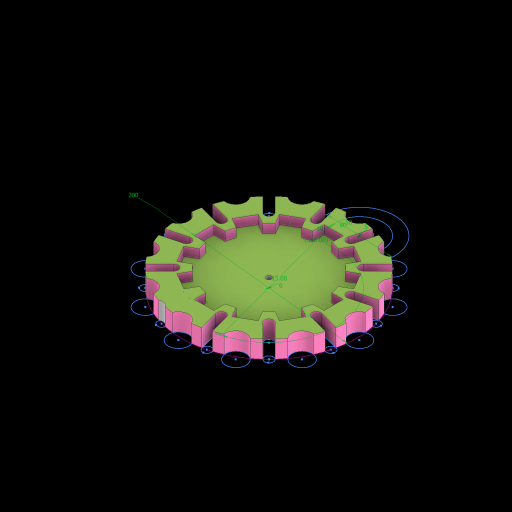
# Autodesk Inventor part: Geneva Gear 12
Saved by Autodesk Inventor 2023 (Build 270158000, 158)
## iProperties
Created: 2022-10-22
Part Number: Geneva Gear 12
Material: Generic
Document SubType Name: Modeling
Designer: annah
Density: 1 g/cm^3
Appearance: Default
Author: annah
Autodesk Inventor part; units mm, degrees
ref_plane "YZ Plane" through (0, 0, 0) normal (1, 0, 0) x (0, 1, 0)
ref_plane "XZ Plane" through (0, 0, 0) normal (0, 1, 0) x (-1, 0, 0)
ref_plane "XY Plane" through (0, 0, 0) normal (0, 0, 1) x (1, 0, 0)
sketch "Sketch1" plane through (0, 0, 0) normal (0, 1, 0) x (-1, 0, 0)
  line L0 (19.134172, -46.193977) -> (0, -54.123064)
  line L1 (0, -54.123064) -> (0, 0)
  line L2 (0, 0) -> (19.134172, -46.193977)
  circle A0 centre (0, 0) radius 50
  line L3 (17.249136, -28.614096) -> (23.883792, -44.631571)
  circle A1 centre (0, -54.123064) radius 20.712
  arc A2 (17.535481, -29.305393) -> (8.166463, -32.781215) centre (12.785861, -30.867798) ccw
  line L4 (14.515069, -48.108105) -> (8.166463, -32.781215)
  line L5 (19.134172, -41.193977) -> (0, -41.193977)
  circle A3 centre (0, -54.123064) radius 12.929087
  arc A4 (-11.696069, -48.612776) -> (11.696069, -48.612776) centre (0, 0) ccw
  arc A5 (-11.696069, -48.612776) -> (11.696069, -48.612776) centre (0, -54.123064) ccw
  circle A6 centre (0, -54.123064) radius 32.5
  arc A7 (19.134172, -41.193977) -> (16.676498, -41.839687) centre (19.134172, -46.193977) ccw
  arc A8 (14.424881, -47.874031) -> (23.597447, -43.940275) centre (19.134172, -46.193977) ccw
  line L6 (32.430202, -8.03624) -> (48.447678, -14.670896)
  arc A9 (33.1215, -8.322585) -> (28.954381, -17.405258) centre (30.867798, -12.785861) ccw
  line L7 (44.281271, -23.753864) -> (28.954381, -17.405258)
  arc A10 (44.051983, -23.652121) -> (47.756382, -14.384552) centre (46.193977, -19.134172) ccw
  circle A11 centre (38.270785, -38.270785) radius 12.929087
  line L8 (28.614096, 17.249136) -> (44.631571, 23.883792)
  arc A12 (29.305393, 17.535481) -> (32.781215, 8.166463) centre (30.867798, 12.785861) ccw
  line L9 (48.108105, 14.515069) -> (32.781215, 8.166463)
  arc A13 (47.874031, 14.424881) -> (43.940275, 23.597447) centre (46.193977, 19.134172) ccw
  circle A14 centre (54.123064, 0) radius 12.929087
  line L10 (8.03624, 32.430202) -> (14.670896, 48.447678)
  arc A15 (8.322585, 33.1215) -> (17.405258, 28.954381) centre (12.785861, 30.867798) ccw
  line L11 (23.753864, 44.281271) -> (17.405258, 28.954381)
  arc A16 (23.652121, 44.051983) -> (14.384552, 47.756382) centre (19.134172, 46.193977) ccw
  circle A17 centre (38.270785, 38.270785) radius 12.929087
  line L12 (-17.249136, 28.614096) -> (-23.883792, 44.631571)
  arc A18 (-17.535481, 29.305393) -> (-8.166463, 32.781215) centre (-12.785861, 30.867798) ccw
  line L13 (-14.515069, 48.108105) -> (-8.166463, 32.781215)
  arc A19 (-14.424881, 47.874031) -> (-23.597447, 43.940275) centre (-19.134172, 46.193977) ccw
  circle A20 centre (0, 54.123064) radius 12.929087
  line L14 (-32.430202, 8.03624) -> (-48.447678, 14.670896)
  arc A21 (-33.1215, 8.322585) -> (-28.954381, 17.405258) centre (-30.867798, 12.785861) ccw
  line L15 (-44.281271, 23.753864) -> (-28.954381, 17.405258)
  arc A22 (-44.051983, 23.652121) -> (-47.756382, 14.384552) centre (-46.193977, 19.134172) ccw
  circle A23 centre (-38.270785, 38.270785) radius 12.929087
  line L16 (-28.614096, -17.249136) -> (-44.631571, -23.883792)
  arc A24 (-29.305393, -17.535481) -> (-32.781215, -8.166463) centre (-30.867798, -12.785861) ccw
  line L17 (-48.108105, -14.515069) -> (-32.781215, -8.166463)
  arc A25 (-47.874031, -14.424881) -> (-43.940275, -23.597447) centre (-46.193977, -19.134172) ccw
  circle A26 centre (-54.123064, 0) radius 12.929087
  line L18 (-8.03624, -32.430202) -> (-14.670896, -48.447678)
  arc A27 (-8.322585, -33.1215) -> (-17.405258, -28.954381) centre (-12.785861, -30.867798) ccw
  line L19 (-23.753864, -44.281271) -> (-17.405258, -28.954381)
  arc A28 (-23.652121, -44.051983) -> (-14.384552, -47.756382) centre (-19.134172, -46.193977) ccw
  circle A29 centre (-38.270785, -38.270785) radius 12.929087
  circle A30 centre (0, 0) radius 3.5
  circle A31 centre (0, -54.123064) radius 3.5
  arc A32 (-7.5, -54.123064) -> (7.5, -54.123064) centre (0, -54.123064) ccw
  arc A33 (7.5, 0) -> (-7.5, 0) centre (0, 0) ccw
  line L20 (7.5, 0) -> (7.5, -54.123064)
  line L21 (-7.5, 0) -> (-7.5, -54.123064)
  circle A34 centre (0, -33.411064) radius 5
  point P0 (8.166168, -32.780503)
  point P1 (23.597447, -43.940275)
  point P2 (28.953669, -17.404963)
  point P3 (29.12854, -29.12854)
  point P4 (26.104054, -42.644793)
  point P5 (42.644793, -26.104054)
  point P6 (32.780503, 8.166168)
  point P7 (41.193977, 0)
  point P8 (48.612776, -11.696069)
  point P9 (48.612776, 11.696069)
  point P10 (17.404963, 28.953669)
  point P11 (29.12854, 29.12854)
  point P12 (42.644793, 26.104054)
  point P13 (26.104054, 42.644793)
  point P14 (-8.166168, 32.780503)
  point P15 (0, 41.193977)
  point P16 (11.696069, 48.612776)
  point P17 (-11.696069, 48.612776)
  point P18 (-28.953669, 17.404963)
  point P19 (-29.12854, 29.12854)
  point P20 (-26.104054, 42.644793)
  point P21 (-42.644793, 26.104054)
  point P22 (-32.780503, -8.166168)
  point P23 (-41.193977, 0)
  point P24 (-48.612776, 11.696069)
  point P25 (-48.612776, -11.696069)
  point P26 (-17.404963, -28.953669)
  point P27 (-29.12854, -29.12854)
  point P28 (-42.644793, -26.104054)
  point P29 (-26.104054, -42.644793)
  point P30 (23.652121, -44.051983)
  point P31 (26.104054, -42.644793)
  point P32 (42.644793, -26.104054)
  point P33 (44.049009, -23.657658)
  point P34 (47.874031, -14.424881)
  point P35 (48.612776, -11.696069)
  point P36 (48.612776, 11.696069)
  point P37 (47.875844, 14.418863)
  point P38 (44.051983, 23.652121)
  point P39 (42.644793, 26.104054)
  point P40 (26.104054, 42.644793)
  point P41 (23.657658, 44.049009)
  point P42 (14.424881, 47.874031)
  point P43 (11.696069, 48.612776)
  point P44 (-11.696069, 48.612776)
  point P45 (-14.418863, 47.875844)
  point P46 (-23.652121, 44.051983)
  point P47 (-26.104054, 42.644793)
  point P48 (-42.644793, 26.104054)
  point P49 (-44.049009, 23.657658)
  point P50 (-47.874031, 14.424881)
  point P51 (-48.612776, 11.696069)
  point P52 (-48.612776, -11.696069)
  point P53 (-47.875844, -14.418863)
  point P54 (-44.051983, -23.652121)
  point P55 (-42.644793, -26.104054)
  point P56 (-26.104054, -42.644793)
  point P57 (-23.657658, -44.049009)
  point P58 (-14.424881, -47.874031)
  point P59 (14.418863, -47.875844)
  dimension "d2" = 100
  dimension "d3" = 22.5
  dimension "d4" = 20.712
  dimension "d5" = 50
  dimension "d6" = 54.12306
  dimension "d7" = 10
  dimension "d8" = 25.85817
  dimension "d9" = 65
  dimension "d10" = 360
  dimension "d11" = 7
  dimension "d12" = 7
  dimension "d13" = 15
  dimension "d14" = 15
  dimension "d15" = 10
  constraints: 113 point on circle, 44 end point, 35 centre point, 28 point on line, 9 coincident, 3 tangent, 2 vertical, 1 concentric, 1 parallel, 1 perpendicular, 161 other
  measures "d2" diameter of A0
  measures "d3" angle of L2 L1
  measures "d4" distance of L0.start L0.end
  measures "d5" distance of L1.end L0.start
  measures "d6" distance of L0.end L1.end
  measures "d7" diameter of A2
  measures "d8" diameter of A3
  measures "d9" diameter of A6
  measures "d11" diameter of A30
  measures "d12" diameter of A31
  measures "d13" diameter of A32
  measures "d14" diameter of A33
  measures "d15" diameter of A34
sketch "Sketch2" plane through (0, 0, 0) normal (0, 1, 0) x (-1, 0, 0)
  circle A0 centre (0, 0) radius 100
  line L0 (0, 0) -> (18.565789, -69.288466)
  line L1 (0, 0) -> (0, -103.527618)
  arc A1 (24.644787, -72.667335) -> (14.990656, -75.254151) centre (0, 0) ccw
  circle A2 centre (25.881905, -96.592583) radius 5
  arc A3 (24.729005, -72.981583) -> (15.074653, -75.567772) centre (19.859884, -74.118095) ccw
  line L2 (30.677672, -95.178151) -> (24.644787, -72.667335)
  line L3 (21.052275, -97.886678) -> (14.990656, -75.254151)
  circle A4 centre (0, -103.527618) radius 11.622857
  line L4 (21.052275, -97.886678) -> (25.881905, -96.592583)
  arc A5 (-25.881905, -96.592583) -> (26.719744, -101.521885) centre (0, -103.527618) ccw
  circle A6 centre (0, -103.527618) radius 40
  arc A7 (57.906738, -50.839403) -> (50.838918, -57.906284) centre (54.258212, -54.258212) ccw
  line L5 (67.175144, -74.246212) -> (50.609365, -57.676679)
  line L6 (74.156719, -67.087861) -> (57.676679, -50.609365)
  circle A8 centre (70.710678, -70.710678) radius 5
  circle A9 centre (51.763809, -89.657547) radius 11.622857
  arc A10 (75.568408, -15.074845) -> (72.980936, -24.728854) centre (74.118095, -19.859884) ccw
  line L7 (95.298487, -30.711534) -> (72.667335, -24.644787)
  line L8 (97.765533, -21.021432) -> (75.254151, -14.990656)
  circle A11 centre (96.592583, -25.881905) radius 5
  circle A12 centre (89.657547, -51.763809) radius 11.622857
  arc A13 (72.981583, 24.729005) -> (75.567772, 15.074653) centre (74.118095, 19.859884) ccw
  line L9 (97.886678, 21.052275) -> (75.254151, 14.990656)
  line L10 (95.178151, 30.677672) -> (72.667335, 24.644787)
  circle A14 centre (96.592583, 25.881905) radius 5
  circle A15 centre (103.527618, 0) radius 11.622857
  arc A16 (50.839403, 57.906738) -> (57.906284, 50.838918) centre (54.258212, 54.258212) ccw
  line L11 (74.246212, 67.175144) -> (57.676679, 50.609365)
  line L12 (67.087861, 74.156719) -> (50.609365, 57.676679)
  circle A17 centre (70.710678, 70.710678) radius 5
  circle A18 centre (89.657547, 51.763809) radius 11.622857
  arc A19 (15.074845, 75.568408) -> (24.728854, 72.980936) centre (19.859884, 74.118095) ccw
  line L13 (30.711534, 95.298487) -> (24.644787, 72.667335)
  line L14 (21.021432, 97.765533) -> (14.990656, 75.254151)
  circle A20 centre (25.881905, 96.592583) radius 5
  circle A21 centre (51.763809, 89.657547) radius 11.622857
  arc A22 (-24.729005, 72.981583) -> (-15.074653, 75.567772) centre (-19.859884, 74.118095) ccw
  line L15 (-21.052275, 97.886678) -> (-14.990656, 75.254151)
  line L16 (-30.677672, 95.178151) -> (-24.644787, 72.667335)
  circle A23 centre (-25.881905, 96.592583) radius 5
  circle A24 centre (0, 103.527618) radius 11.622857
  arc A25 (-57.906738, 50.839403) -> (-50.838918, 57.906284) centre (-54.258212, 54.258212) ccw
  line L17 (-67.175144, 74.246212) -> (-50.609365, 57.676679)
  line L18 (-74.156719, 67.087861) -> (-57.676679, 50.609365)
  circle A26 centre (-70.710678, 70.710678) radius 5
  circle A27 centre (-51.763809, 89.657547) radius 11.622857
  arc A28 (-75.568408, 15.074845) -> (-72.980936, 24.728854) centre (-74.118095, 19.859884) ccw
  line L19 (-95.298487, 30.711534) -> (-72.667335, 24.644787)
  line L20 (-97.765533, 21.021432) -> (-75.254151, 14.990656)
  circle A29 centre (-96.592583, 25.881905) radius 5
  circle A30 centre (-89.657547, 51.763809) radius 11.622857
  arc A31 (-72.981583, -24.729005) -> (-75.567772, -15.074653) centre (-74.118095, -19.859884) ccw
  line L21 (-97.886678, -21.052275) -> (-75.254151, -14.990656)
  line L22 (-95.178151, -30.677672) -> (-72.667335, -24.644787)
  circle A32 centre (-96.592583, -25.881905) radius 5
  circle A33 centre (-103.527618, 0) radius 11.622857
  arc A34 (-50.839403, -57.906738) -> (-57.906284, -50.838918) centre (-54.258212, -54.258212) ccw
  line L23 (-74.246212, -67.175144) -> (-57.676679, -50.609365)
  line L24 (-67.087861, -74.156719) -> (-50.609365, -57.676679)
  circle A35 centre (-70.710678, -70.710678) radius 5
  circle A36 centre (-89.657547, -51.763809) radius 11.622857
  arc A37 (-15.074845, -75.568408) -> (-24.728854, -72.980936) centre (-19.859884, -74.118095) ccw
  line L25 (-30.711534, -95.298487) -> (-24.644787, -72.667335)
  line L26 (-21.021432, -97.765533) -> (-14.990656, -75.254151)
  circle A38 centre (-25.881905, -96.592583) radius 5
  circle A39 centre (-51.763809, -89.657547) radius 11.622857
  circle A40 centre (0, 0) radius 3
  circle A41 centre (0, -103.527618) radius 2.5
  point P0 (50.722678, -50.722678)
  point P1 (73.90092, -74.56066)
  point P2 (69.288466, -18.565789)
  point P3 (101.280404, -27.620965)
  point P4 (69.288466, 18.565789)
  point P5 (101.521885, 26.719744)
  point P6 (50.722678, 50.722678)
  point P7 (74.56066, 73.90092)
  point P8 (18.565789, 69.288466)
  point P9 (27.620965, 101.280404)
  point P10 (-18.565789, 69.288466)
  point P11 (-26.719744, 101.521885)
  point P12 (-50.722678, 50.722678)
  point P13 (-73.90092, 74.56066)
  point P14 (-69.288466, 18.565789)
  point P15 (-101.280404, 27.620965)
  point P16 (-69.288466, -18.565789)
  point P17 (-101.521885, -26.719744)
  point P18 (-50.722678, -50.722678)
  point P19 (-74.56066, -73.90092)
  point P20 (-18.565789, -69.288466)
  point P21 (-27.620965, -101.280404)
  point P22 (40.291734, -91.523637)
  point P23 (59.115928, -80.655484)
  point P24 (67.086711, -74.157759)
  point P25 (80.655484, -59.115928)
  point P26 (91.523637, -40.291734)
  point P27 (95.177675, -30.679148)
  point P28 (99.407662, -10.868153)
  point P29 (99.407662, 10.868153)
  point P30 (97.765859, 21.019917)
  point P31 (91.523637, 40.291734)
  point P32 (80.655484, 59.115928)
  point P33 (74.157759, 67.086711)
  point P34 (59.115928, 80.655484)
  point P35 (40.291734, 91.523637)
  point P36 (30.679148, 95.177675)
  point P37 (10.868153, 99.407662)
  point P38 (-10.868153, 99.407662)
  point P39 (-21.019917, 97.765859)
  point P40 (-40.291734, 91.523637)
  point P41 (-59.115928, 80.655484)
  point P42 (-67.086711, 74.157759)
  point P43 (-80.655484, 59.115928)
  point P44 (-91.523637, 40.291734)
  point P45 (-95.177675, 30.679148)
  point P46 (-99.407662, 10.868153)
  point P47 (-99.407662, -10.868153)
  point P48 (-97.765859, -21.019917)
  point P49 (-91.523637, -40.291734)
  point P50 (-80.655484, -59.115928)
  point P51 (-74.157759, -67.086711)
  point P52 (-59.115928, -80.655484)
  point P53 (-40.291734, -91.523637)
  point P54 (-30.679148, -95.177675)
  point P55 (-10.868153, -99.407662)
  point P56 (10.868153, -99.407662)
  point P57 (21.019917, -97.765859)
  dimension "d16" = 200
  dimension "d17" = 15
  dimension "d20" = 10
  dimension "d21" = 10
  dimension "d22" = 80
  dimension "d25" = 360
  dimension "d27" = 6
  dimension "d28" = 5
  constraints: 100 point on circle, 54 end point, 41 centre point, 25 point on line, 8 coincident, 1 vertical, 198 other
  measures "d17" angle of L1 L0
  measures "d20" diameter of A2
  measures "d21" diameter of A3
  measures "d22" diameter of A6
  measures "d27" diameter of A40
  measures "d28" diameter of A41
extrude "Extrusion1" add sketch "Sketch2" along normal blind 20 contours L26 A37 A1 L1 A4 A0 | A0 A6 A1 A37 L25 | A0 A39 L24 A34 A1 A6 | L1 A1 A3 L3 A0 A4 | A37 A6 L1 A1 | A6 A37 A1 | A1 A34 A31 A28 A25 A22 A19 A16 A13 A10 A7 A6 A3 L0 A40 L1 A37 | L1 A6 L0 A3 A1 | A6 A1 A7 L5 A0 A9 | A0 L2 A3 A1 A6 | L1 A40 L0 A6 | A34 L23 A0 A36 L22 A31 A1 | A1 A3 A6 | A6 A3 L0 | A31 L21 A0 A33 L20 A28 A1 | A1 A10 L7 A0 A12 L6 A7 | A28 L19 A0 A30 L18 A25 A1 | A1 A13 L9 A0 A15 L8 A10 | A25 L17 A0 A27 L16 A22 A1 | A1 A16 L11 A0 A18 L10 A13 | A22 L15 A0 A24 L14 A19 A1 | A1 A19 L13 A0 A21 L12 A16 picked at (-24.752418, -72.385942)
sketch "Sketch3" plane through (0, 20, 0) normal (0, 1, 0) x (1, 0, 0)
  circle A0 centre (0, 0) radius 3
  line L0 (-11.003106, 74.096865) -> (11.003106, 74.096865)
  line L1 (11.003106, 74.096865) -> (11.003106, 56.269048)
  line L2 (11.003106, 56.269048) -> (-11.003106, 56.269048)
  line L3 (-11.003106, 56.269048) -> (-11.003106, 74.096865)
  line L4 (11.003106, 74.096865) -> (0, 65.182957) construction
  line L5 (-27.519463, 69.671321) -> (-18.605555, 54.231978)
  line L6 (-18.605555, 54.231978) -> (-37.663494, 43.228872)
  line L7 (-37.663494, 43.228872) -> (-46.577402, 58.668215)
  line L8 (-46.577402, 58.668215) -> (-27.519463, 69.671321)
  line L9 (-58.668215, 46.577402) -> (-43.228872, 37.663494)
  line L10 (-43.228872, 37.663494) -> (-54.231978, 18.605555)
  line L11 (-54.231978, 18.605555) -> (-69.671321, 27.519463)
  line L12 (-69.671321, 27.519463) -> (-58.668215, 46.577402)
  line L13 (-74.096865, 11.003106) -> (-56.269048, 11.003106)
  line L14 (-56.269048, 11.003106) -> (-56.269048, -11.003106)
  line L15 (-56.269048, -11.003106) -> (-74.096865, -11.003106)
  line L16 (-74.096865, -11.003106) -> (-74.096865, 11.003106)
  line L17 (-69.671321, -27.519463) -> (-54.231978, -18.605555)
  line L18 (-54.231978, -18.605555) -> (-43.228872, -37.663494)
  line L19 (-43.228872, -37.663494) -> (-58.668215, -46.577402)
  line L20 (-58.668215, -46.577402) -> (-69.671321, -27.519463)
  line L21 (-46.577402, -58.668215) -> (-37.663494, -43.228872)
  line L22 (-37.663494, -43.228872) -> (-18.605555, -54.231978)
  line L23 (-18.605555, -54.231978) -> (-27.519463, -69.671321)
  line L24 (-27.519463, -69.671321) -> (-46.577402, -58.668215)
  line L25 (-11.003106, -74.096865) -> (-11.003106, -56.269048)
  line L26 (-11.003106, -56.269048) -> (11.003106, -56.269048)
  line L27 (11.003106, -56.269048) -> (11.003106, -74.096865)
  line L28 (11.003106, -74.096865) -> (-11.003106, -74.096865)
  line L29 (27.519463, -69.671321) -> (18.605555, -54.231978)
  line L30 (18.605555, -54.231978) -> (37.663494, -43.228872)
  line L31 (37.663494, -43.228872) -> (46.577402, -58.668215)
  line L32 (46.577402, -58.668215) -> (27.519463, -69.671321)
  line L33 (58.668215, -46.577402) -> (43.228872, -37.663494)
  line L34 (43.228872, -37.663494) -> (54.231978, -18.605555)
  line L35 (54.231978, -18.605555) -> (69.671321, -27.519463)
  line L36 (69.671321, -27.519463) -> (58.668215, -46.577402)
  line L37 (74.096865, -11.003106) -> (56.269048, -11.003106)
  line L38 (56.269048, -11.003106) -> (56.269048, 11.003106)
  line L39 (56.269048, 11.003106) -> (74.096865, 11.003106)
  line L40 (74.096865, 11.003106) -> (74.096865, -11.003106)
  line L41 (69.671321, 27.519463) -> (54.231978, 18.605555)
  line L42 (54.231978, 18.605555) -> (43.228872, 37.663494)
  line L43 (43.228872, 37.663494) -> (58.668215, 46.577402)
  line L44 (58.668215, 46.577402) -> (69.671321, 27.519463)
  line L45 (46.577402, 58.668215) -> (37.663494, 43.228872)
  line L46 (37.663494, 43.228872) -> (18.605555, 54.231978)
  line L47 (18.605555, 54.231978) -> (27.519463, 69.671321)
  line L48 (27.519463, 69.671321) -> (46.577402, 58.668215)
  arc A1 (-11.003106, 60.9667) -> (-20.954381, 58.300264) centre (0, 0) ccw
  arc A2 (20.954381, 58.300264) -> (11.003106, 60.9667) centre (0, 0) ccw
  arc A3 (47.297158, 40.01232) -> (40.01232, 47.297158) centre (0, 0) ccw
  arc A4 (-40.01232, 47.297158) -> (-47.297158, 40.01232) centre (0, 0) ccw
  arc A5 (-58.300264, 20.954381) -> (-60.9667, 11.003106) centre (0, 0) ccw
  arc A6 (-60.9667, -11.003106) -> (-58.300264, -20.954381) centre (0, 0) ccw
  arc A7 (-47.297158, -40.01232) -> (-40.01232, -47.297158) centre (0, 0) ccw
  arc A8 (-20.954381, -58.300264) -> (-11.003106, -60.9667) centre (0, 0) ccw
  arc A9 (11.003106, -60.9667) -> (20.954381, -58.300264) centre (0, 0) ccw
  arc A10 (40.01232, -47.297158) -> (47.297158, -40.01232) centre (0, 0) ccw
  arc A11 (58.300264, -20.954381) -> (60.9667, -11.003106) centre (0, 0) ccw
  arc A12 (60.9667, 11.003106) -> (58.300264, 20.954381) centre (0, 0) ccw
  dimension "d36" = 360
  constraints: 98 end point, 24 point on circle, 24 point on line, 12 centre point, 3 coincident, 2 parallel, 1 horizontal, 1 perpendicular, 97 other
extrude "Extrusion2" cut sketch "Sketch3" against normal blind 10
extrude "Extrusion3" add sketch "Sketch2" along normal blind 20 contours L14 A20 L13 A1 | A1 A19 | A0 A20
sketch "Sketch4" plane through (0, 20, 0) normal (0, 1, 0) x (1, 0, 0)
  arc A0 (-40.291734, -91.523637) -> (-10.868153, -99.407662) centre (0, 0) ccw
  arc A1 (-20.910837, -97.789247) -> (-30.655137, -95.185412) centre (-27.010133, -101.079661) ccw
  constraints: 4 point on circle, 1 centre point
extrude "Extrusion4" cut sketch "Sketch4" against normal blind 20
body "Solid1"
